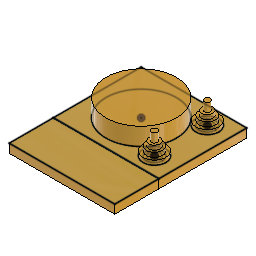
azimuth motor v6 (Autodesk Fusion 360 design; units mm, degrees)
Autodesk Fusion 360 part; units mm, degrees
sketch "Sketch1" plane through (0, 0, 0) normal (0, 0, 1) x (1, 0, 0)
  circle A0 centre (0, 0) radius 2
  line L0 (-2.5, -2.5) -> (3.5, -2.5)
  line L1 (3.5, -2.5) -> (3.5, 2.5)
  line L2 (3.5, 2.5) -> (-2.5, 2.5)
  line L3 (-2.5, 2.5) -> (-2.5, -2.5)
  circle A1 centre (2.2522, -1.4961) radius 0.65
  circle A2 centre (2.2522, 1.5092) radius 0.65
  circle A3 centre (2.2522, 1.5092) radius 0.4628
  circle A4 centre (2.2522, 1.5092) radius 0.3128
  circle A5 centre (2.2522, 1.5092) radius 0.1684
  circle A6 centre (2.2522, -1.4961) radius 0.4628
  circle A7 centre (2.2522, -1.4961) radius 0.3128
  circle A8 centre (2.2522, -1.4961) radius 0.1684
  line L4 (-2.5, -2.5) -> (3.5, -2.5)
  line L5 (3.5, -2.5) -> (3.5, -5)
  line L6 (3.5, -5) -> (-2.5, -5)
  line L7 (-2.5, -5) -> (-2.5, -2.5)
  dimension "d1" = 4
  dimension "d2" = 1.3
  dimension "d3" = 1.3
  dimension "d20" = 2.5
  dimension "d21" = 5
  dimension "d22" = 6
  dimension "d23" = 2.5
  dimension "d24" = 5
  dimension "d25" = 6
  dimension "d26" = 1.2478
  dimension "d27" = 1.2478
  dimension "d28" = 0.9908
  dimension "d29" = 1.0039
  dimension "d30" = 2.5
  dimension "d31" = 2.5
  dimension "d32" = 0.9255
  dimension "d33" = 0.6255
  dimension "d34" = 0.3367
  constraint coincident A0.centre origin
  constraint concentric A2 A3
  constraint concentric A2 A4
  constraint concentric A4 A5
  constraint concentric A1 A6
  constraint concentric A1 A7
  constraint concentric A1 A8
  constraint horizontal L6
  constraint vertical L7
  constraint vertical L5
  constraint vertical L1
  constraint equal A3 A6
  constraint equal A4 A7
  constraint equal A5 A8
  measures "d1" diameter of A0
  measures "d2" diameter of A1
  measures "d3" diameter of A2
  measures "d20" distance of L0.start L6.end
  measures "d21" distance of L0.start L2.end
  measures "d22" distance of L1.end L2.end
  measures "d23" distance of L0.end L5.end
  measures "d24" distance of L0.end L1.end
  measures "d25" distance of L0.start L0.end
  measures "d26" distance of L1 A2.centre
  measures "d27" distance of L1 A1.centre
  measures "d28" distance of L2 A2.centre
  measures "d29" distance of L0 A1.centre
  measures "d30" distance of A0.centre L3
  measures "d31" distance of A0.centre L2
  measures "d32" diameter of A3
  measures "d33" diameter of A4
  measures "d34" diameter of A5
extrude "Extrude9" add sketch "Sketch1" along normal blind 0.25 contours A1 | A2 makes body 1 at (2.9014, -1.5285, 0.1667) makes body 2 at (2.9014, 1.4768, 0.1667)
extrude "Extrude8" add sketch "Sketch1" against normal blind 0.5 separate body contours L0 L1 L2 L3 L4 | L0 L4 L5 L6 L7 makes body 3
extrude "Extrude10" add sketch "Sketch1" along normal blind 0.5 contours A3 | A6 bodies 1 2 3
extrude "Extrude11" add sketch "Sketch1" along normal blind 0.75 contours A4 | A7 bodies 1 2 3
extrude "Extrude12" add sketch "Sketch1" along normal blind 1.25 contours A5 | A8 bodies 1 2 3
extrude "Extrude13" add sketch "Sketch1" against normal blind 0.5 contours A1 | A2 | A3 | A4 | A5 | A6 | A7 | A8 bodies 1 2 3
extrude "Extrude14" add sketch "Sketch1" against normal blind 0.5 contours A0 bodies 1
extrude "Extrude15" add sketch "Sketch1" along normal blind 1 contours A0 bodies 1
extrude "Extrude2" [suppressed]
extrude "Extrude1" [suppressed]
extrude "Extrude3" [suppressed]
extrude "Extrude4" [suppressed]
extrude "Extrude5" [suppressed]
extrude "Extrude6" [suppressed]
extrude "Extrude7" [suppressed]
